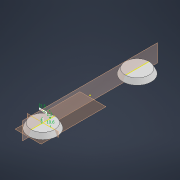
# Autodesk Inventor part: 手把
Saved by Autodesk Inventor 2022 (Build 260153000, 153)
## iProperties
Created: 2022-04-22
Part Number: 手把
Material: 一般
Document SubType Name: Modeling
Designer: User
Density: 1 g/cm^3
Appearance: 預設
Author: User
Autodesk Inventor part; units mm, degrees
sketch "草圖1" plane through (0, 0, 0) normal (0, 1, 0) x (-1, 0, 0)
  circle A0 centre (0, 50) radius 12.5
  point P0 (0, 0)
  dimension "d0" = 25
  dimension "d1" = 50
  constraints: 1 centre point, 1 vertical alignment
  measures "d0" diameter of A0
  measures "d1" distance of point (0, 0) A0.centre
ref_plane "工作平面1" through (0, -5, 0) normal (0, 1, 0) x (-1, 0, 0)
sketch "草圖2" plane through (0, -5, 0) normal (0, 1, 0) x (-1, 0, 0)
  circle A0 centre (0, 50) radius 15
  point P0 (0, 0)
  dimension "d3" = 30
  constraints: 1 centre point, 1 coincident
  measures "d3" diameter of A0
loft "斷面混成1" add profiles "草圖2", "草圖1"
mirror "鏡射1" about plane through (0, 0, 0) normal (0, 0, 1)
ref_plane "工作平面2" through (0, 0, 50) normal (0, 0, 1) x (1, 0, 0)
sketch "草圖3" plane through (0, 0, 50) normal (0, 0, 1) x (1, 0, 0)
  line L0 (-3.75, 10.6) -> (3.75, 10.6)
  line L1 (3.75, 10.6) -> (3.75, 11.8)
  line L2 (3.75, 11.8) -> (-3.75, 11.8)
  line L3 (-3.75, 11.8) -> (-3.75, 10.6)
  line L4 (-12.5, 0) -> (12.5, 0) projected
  point P0 (0, 0)
  point P1 (0, 10.6)
  dimension "d9" = 7.5
  dimension "d10" = 1.2
  dimension "d11" = 10.6
  constraints: 8 end point, 2 parallel, 1 horizontal, 1 midpoint, 1 perpendicular, 1 vertical alignment
  measures "d9" distance of L2.end L1.end
  measures "d10" distance of L1.end L0.end
  measures "d11" distance from line of L4 point (0, 10.6)
sketch "草圖4" plane through (0, 0, 0) normal (1, 0, 0) x (0, 1, 0)
  line L0 (10.6, 50) -> (11.8, 50) projected
  line L1 (0, 62.5) -> (0, 37.5) projected
  line L2 (0, -62.5) -> (0, -37.5) projected
  line L3 (0, 50) -> (5, 50)
  point P0 (0, 0)
  dimension "d12" = 5
  constraints: 2 end point, 1 horizontal, 1 midpoint
  measures "d12" distance of L3.start L3.end
